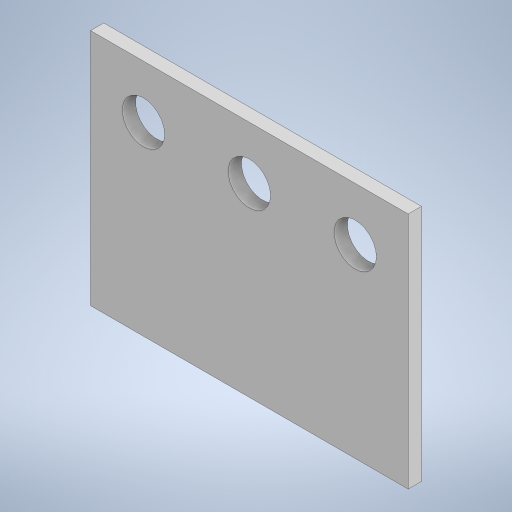
# Autodesk Inventor part: flatPoly3ForCNC
Saved by Autodesk Inventor 2023.4 (Build 274418000, 418)
## iProperties
Created: 2023-12-19
Part Number: flatPoly3ForCNC
Material: Generic
Document SubType Name: Modeling
Designer: Meer
Density: 1 g/cm^3
Appearance: Default
Author: Meer
Autodesk Inventor part; units mm, degrees
ref_plane "YZ Plane" through (0, 0, 0) normal (1, 0, 0) x (0, 1, 0)
ref_plane "XZ Plane" through (0, 0, 0) normal (0, 1, 0) x (-1, 0, 0)
ref_plane "XY Plane" through (0, 0, 0) normal (0, 0, 1) x (1, 0, 0)
sketch "Sketch1" plane through (0, 0, 0) normal (0, 0, 1) x (1, 0, 0)
  line L0 (0, 0) -> (38.1, 0)
  line L1 (38.1, 0) -> (38.1, 28.575)
  line L2 (38.1, 28.575) -> (0, 28.575)
  line L3 (0, 28.575) -> (0, 0)
  circle A0 centre (6.35, 22.225) radius 2.54
  circle A1 centre (19.05, 22.225) radius 2.54
  circle A2 centre (31.75, 22.225) radius 2.54
  dimension "d0" = 38.1
  dimension "d1" = 28.575
  dimension "d5" = 5.08
  dimension "d8" = 5.08
  dimension "d9" = 5.08
  constraints: 8 end point, 3 centre point, 2 parallel, 1 horizontal, 1 perpendicular
  measures "d0" distance of L2.end L1.end
  measures "d1" distance of L0.end L1.end
  measures "d5" diameter of A0
  measures "d8" diameter of A1
  measures "d9" diameter of A2
extrude "Extrusion1" add sketch "Sketch1" along normal blind 1.5875
body "Solid1"
